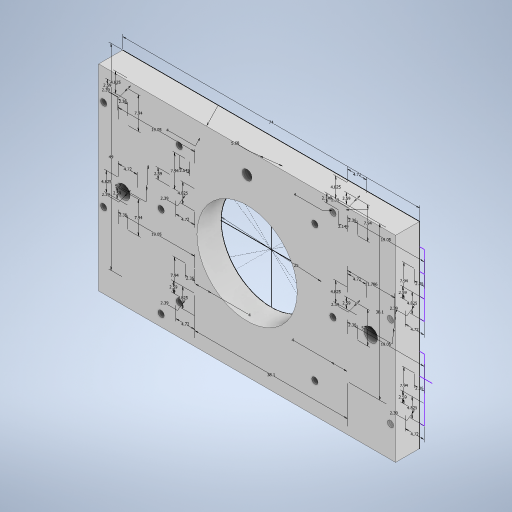
# Autodesk Inventor part: adapter-plate
Saved by Autodesk Inventor 2024 (Build 280153000, 153)
## iProperties
Created: 2023-08-30
Part Number: adapter-plate
Material: Generic
Document SubType Name: Modeling
Designer: raad
Density: 1 g/cm^3
Appearance: Default
Author: raad
Autodesk Inventor part; units mm, degrees
ref_plane "YZ Plane" through (0, 0, 0) normal (1, 0, 0) x (0, 1, 0)
ref_plane "XZ Plane" through (0, 0, 0) normal (0, 1, 0) x (-1, 0, 0)
ref_plane "XY Plane" through (0, 0, 0) normal (0, 0, 1) x (1, 0, 0)
sketch "Sketch1" plane through (0, 0, 0) normal (0, 0, 1) x (1, 0, 0)
  line L0 (37, -24.5) -> (-37, -24.5)
  line L1 (-37, -24.5) -> (-37, 24.5)
  line L2 (-37, 24.5) -> (37, 24.5)
  line L3 (37, 24.5) -> (37, -24.5)
  line L4 (37, -24.5) -> (-37, 24.5) construction
  line L5 (-37, -24.5) -> (37, 24.5) construction
  circle A0 centre (0, 0) radius 12.5
  line L6 (-19.05, 19.05) -> (19.05, 19.05)
  line L7 (19.05, 19.05) -> (19.05, -19.05)
  line L8 (19.05, -19.05) -> (-19.05, -19.05)
  line L9 (-19.05, -19.05) -> (-19.05, 19.05)
  line L10 (-19.05, 19.05) -> (19.05, -19.05) construction
  line L11 (19.05, 19.05) -> (-19.05, -19.05) construction
  line L12 (19.05, 19.05) -> (16.9012, 19.05)
  line L13 (16.9012, 19.05) -> (16.9012, 16.9012)
  line L14 (16.9012, 16.9012) -> (19.05, 16.9012)
  line L15 (19.05, 16.9012) -> (19.05, 19.05)
  line L16 (0, 19.05) -> (0, -19.05)
  line L17 (-19.05, 0) -> (19.05, 0)
  line L18 (-16.9012, 19.05) -> (-16.9012, 16.9012)
  line L19 (-16.9012, 16.9012) -> (-19.05, 16.9012)
  line L20 (19.05, 0) -> (-19.05, 0)
  line L21 (16.9012, -19.05) -> (16.9012, -16.9012)
  line L22 (16.9012, -16.9012) -> (19.05, -16.9012)
  line L23 (-16.9012, -16.9012) -> (-19.05, -16.9012)
  line L24 (-16.9012, -19.05) -> (-16.9012, -16.9012)
  line L25 (19.05, 0) -> (30.8356, 0)
  line L26 (-19.05, 0) -> (-30.8356, 0)
  circle A1 centre (-16.9012, 16.9012) radius 2
  circle A2 centre (16.9012, 16.9012) radius 2
  circle A3 centre (16.9012, -16.9012) radius 2
  circle A4 centre (-16.9012, -16.9012) radius 2
  circle A5 centre (-30.8356, 0) radius 2.85
  circle A6 centre (30.8356, 0) radius 2.85
  line L27 (-30.8356, 14.9012) -> (-30.8356, 2.85)
  line L28 (-38.1003, 8.8756) -> (-19.0503, 8.8756)
  line L29 (-22.8548, 8.8756) -> (-20.3098, 8.8756)
  line L30 (-21.4103, 8.8756) -> (-21.4103, 0.9356)
  line L31 (-38.1719, 10.7443) -> (-35.8119, 10.7443)
  line L32 (-35.7403, 8.8756) -> (-35.7403, 16.8156)
  line L33 (-38.1719, 16.29) -> (-38.1719, 13.7)
  line L34 (-35.7403, 14.2256) -> (-19.0503, 14.2256)
  line L35 (-19.0503, 14.2256) -> (-19.0503, 8.8756)
  line L36 (-25.2148, 0.9356) -> (-25.2148, 3.5256)
  line L37 (-21.4103, 3.5256) -> (-38.1003, 3.5256)
  line L38 (-38.1003, 14.2256) -> (-35.7403, 14.2256)
  line L39 (-21.4103, 3.5256) -> (-19.0503, 3.5256)
  line L40 (-19.0503, 3.5256) -> (-19.0503, 8.8756)
  line L41 (-35.8119, 14.2256) -> (-35.8119, 19.0506)
  line L42 (-38.1003, 19.0506) -> (-33.3803, 19.0506)
  line L43 (-33.3803, 19.0506) -> (-33.3803, 14.2256)
  line L44 (-19.0503, 3.5256) -> (-19.0503, -1.2994)
  line L45 (-19.0503, -1.2994) -> (-23.7703, -1.2994)
  line L46 (-23.7703, -1.2994) -> (-23.7703, 3.5256)
  circle A7 centre (-35.7403, 16.8156) radius 1.195
  circle A8 centre (-21.4103, 0.9356) radius 1.195
  line L47 (30.8356, -2.85) -> (30.8356, -14.9012)
  line L48 (33.9356, -8.8756) -> (40.1, -8.8756)
  line L49 (19.05, -8.8756) -> (38.1, -8.8756)
  line L50 (35.74, -8.8756) -> (35.74, -16.8156)
  line L51 (21.41, -8.8756) -> (21.41, -0.9356)
  line L52 (21.41, -3.5256) -> (38.1, -3.5256)
  line L53 (38.1, -3.5256) -> (38.1, -8.8756)
  line L54 (35.74, -14.2256) -> (19.05, -14.2256)
  line L55 (19.05, -3.5256) -> (21.41, -3.5256)
  line L56 (30.8356, -14.2256) -> (33.1956, -14.2256)
  line L57 (38.1, -14.2256) -> (38.1, -8.8756)
  line L58 (19.05, 1.2994) -> (23.77, 1.2994)
  line L59 (23.77, 1.2994) -> (23.77, -3.5256)
  line L60 (38.1, -14.2256) -> (38.1, -19.0506)
  line L61 (38.1, -19.0506) -> (33.38, -19.0506)
  line L62 (33.38, -19.0506) -> (33.38, -14.2256)
  circle A9 centre (21.41, -0.9356) radius 1.195
  circle A10 centre (35.74, -16.8156) radius 1.195
  line L63 (-38.1, -13.7) -> (-19.05, -13.7)
  line L64 (-21.41, -13.7) -> (-21.41, -21.64)
  line L65 (-35.74, -13.7) -> (-35.74, -5.76)
  line L66 (-35.74, -8.35) -> (-19.05, -8.35)
  line L67 (-19.05, -7.985) -> (-19.05, -13.335)
  line L68 (-21.41, -19.05) -> (-38.1, -19.05)
  line L69 (-38.1, -8.35) -> (-35.74, -8.35)
  line L70 (-21.41, -19.05) -> (-19.05, -19.05)
  line L71 (-19.05, -18.685) -> (-19.05, -13.335)
  line L72 (-38.1, -3.525) -> (-33.38, -3.525)
  line L73 (-33.38, -3.525) -> (-33.38, -8.35)
  line L74 (-19.05, -19.05) -> (-19.05, -23.875)
  line L75 (-19.05, -23.875) -> (-23.77, -23.875)
  line L76 (-23.77, -23.875) -> (-23.77, -19.05)
  circle A11 centre (-35.74, -5.76) radius 1.195
  circle A12 centre (-21.41, -21.64) radius 1.195
  line L77 (19.05, 13.7) -> (38.1, 13.7)
  line L78 (35.74, 13.7) -> (35.74, 5.76)
  line L79 (21.41, 13.7) -> (21.41, 21.64)
  line L80 (21.41, 19.05) -> (38.1, 19.05)
  line L81 (38.1, 19.05) -> (38.1, 13.7)
  line L82 (35.74, 8.35) -> (19.05, 8.35)
  line L83 (19.05, 19.05) -> (21.41, 19.05)
  line L84 (35.74, 8.35) -> (38.1, 8.35)
  line L85 (38.1, 8.35) -> (38.1, 13.7)
  line L86 (19.05, 23.875) -> (23.77, 23.875)
  line L87 (23.77, 23.875) -> (23.77, 19.05)
  line L88 (38.1, 8.35) -> (38.1, 3.525)
  line L89 (38.1, 3.525) -> (33.38, 3.525)
  line L90 (33.38, 3.525) -> (33.38, 8.35)
  circle A13 centre (21.41, 21.64) radius 1.195
  circle A14 centre (35.74, 5.76) radius 1.195
  arc A15 (-37, 21.2315) -> (-36.9905, 20.9193) centre (-31.8628, 21.2315) ccw
  line L91 (-38.1, -3.525) -> (-38.1, -19.05)
  line L92 (19.05, 1.2994) -> (19.05, -14.2256)
  circle A16 centre (0, 19.05) radius 2.84
  dimension "d29" = 5.7
  dimension "d0" = 74
  dimension "d1" = 49
  dimension "d2" = 25
  dimension "d3" = 38.1
  dimension "d4" = 38.1
  dimension "d5" = 2.1488
  dimension "d6" = 2.1488
  dimension "d7" = 11.7856
  dimension "d24" = 4
  dimension "d25" = 4
  dimension "d26" = 4
  dimension "d27" = 4
  dimension "d28" = 5.7
  dimension "d30" = 19.05
  dimension "d31" = 2.545
  dimension "d32" = 7.94
  dimension "d33" = 2.36
  dimension "d34" = 7.94
  dimension "d35" = 2.59
  dimension "d36" = 2.59
  dimension "d37" = 4.825
  dimension "d39" = 4.825
  dimension "d40" = 4.72
  dimension "d41" = 2.39
  dimension "d42" = 2.39
  dimension "d43" = 19.05
  dimension "d44" = 2.36
  dimension "d45" = 7.94
  dimension "d46" = 2.36
  dimension "d47" = 7.94
  dimension "d48" = 2.59
  dimension "d49" = 2.59
  dimension "d50" = 4.825
  dimension "d51" = 4.72
  dimension "d52" = 4.825
  dimension "d53" = 4.72
  dimension "d54" = 2.39
  dimension "d55" = 2.39
  dimension "d56" = 19.05
  dimension "d57" = 2.36
  dimension "d58" = 7.94
  dimension "d59" = 2.36
  dimension "d60" = 7.94
  dimension "d61" = 2.59
  dimension "d62" = 2.59
  dimension "d63" = 4.825
  dimension "d64" = 4.72
  dimension "d65" = 4.825
  dimension "d66" = 4.72
  dimension "d67" = 2.39
  dimension "d68" = 2.39
  dimension "d69" = 19.05
  dimension "d70" = 2.36
  dimension "d71" = 7.94
  dimension "d72" = 2.36
  dimension "d73" = 7.94
  dimension "d74" = 2.59
  dimension "d75" = 2.59
  dimension "d76" = 4.825
  dimension "d77" = 4.72
  dimension "d78" = 4.825
  dimension "d79" = 4.72
  dimension "d80" = 2.39
  dimension "d81" = 2.39
  constraints: 186 end point, 32 point on line, 30 perpendicular, 16 centre point, 16 coincident, 13 symmetric about line, 11 parallel, 8 midpoint, 4 horizontal, 3 vertical, 2 point on circle, 1 tangent, 1 vertical alignment, 2 other
  measures "d0" distance of L1.end L2.end
  measures "d1" distance of L0.end L1.end
  measures "d2" diameter of A0
  measures "d3" distance of L7.end L8.end
  measures "d4" distance of L6.end L7.end
  measures "d5" distance of L14.end L13.end
  measures "d6" distance of L13.end L12.end
  measures "d7" distance of L20.start L25.end
  measures "d24" diameter of A1
  measures "d25" diameter of A2
  measures "d26" diameter of A3
  measures "d27" diameter of A4
  measures "d28" diameter of A5
  measures "d30" distance of L28.start L28.end
  measures "d31" distance of L29.start L29.end
  measures "d32" distance of L30.start L30.end
  measures "d33" distance of L31.start L31.end
  measures "d34" distance of L32.start L32.end
  measures "d35" distance of L33.start L33.end
  measures "d36" distance of L36.start L36.end
  measures "d37" distance of L41.start L41.end
  measures "d39" distance of L39.end L44.end
  measures "d40" distance of L44.end L45.end
  measures "d41" diameter of A7
  measures "d42" diameter of A8
  measures "d43" distance of L49.start L53.end
  measures "d44" distance of L53.end L50.start
  measures "d45" distance of L50.start L50.end
  measures "d46" distance of L49.start L51.start
  measures "d47" distance of L51.start L51.end
  measures "d48" distance of L51.end L52.start
  measures "d49" distance of L50.end L54.start
  measures "d50" distance of L55.start L58.start
  measures "d51" distance of L58.start L58.end
  measures "d52" distance of L57.start L60.end
  measures "d53" distance of L60.end L61.end
  measures "d54" diameter of A9
  measures "d55" diameter of A10
  measures "d56" distance of L63.start L63.end
  measures "d57" distance of L63.end L64.start
  measures "d58" distance of L64.start L64.end
  measures "d59" distance of L63.start L65.start
  measures "d60" distance of L65.start L65.end
  measures "d61" distance of L65.end L66.start
  measures "d62" distance of L64.end L68.start
  measures "d63" distance of L69.start L72.start
  measures "d64" distance of L72.start L72.end
  measures "d65" distance of L74.start L74.end
  measures "d66" distance of L74.end L75.end
  measures "d67" diameter of A11
  measures "d68" diameter of A12
  measures "d69" distance of L77.start L81.end
  measures "d70" distance of L81.end L78.start
  measures "d71" distance of L78.start L78.end
  measures "d72" distance of L77.start L79.start
  measures "d73" distance of L79.start L79.end
  measures "d74" distance of L79.end L80.start
  measures "d75" distance of L78.end L82.start
  measures "d76" distance of L83.start L86.start
  measures "d77" distance of L86.start L86.end
  measures "d78" distance of L85.start L88.end
  measures "d79" distance of L88.end L89.end
  measures "d80" diameter of A13
  measures "d81" diameter of A14
extrude "Extrusion1" add sketch "Sketch1" along normal blind 6 contours L0 L1 L68 L76 L75 L74 L8 L7 L54 L62 L61 L3 | A10 | L61 L62 L54 L50 L48 L3 | L1 L63 L64 L68 | L48 L49 L47 L52 L3 | L1 L69 L65 L63 | A12 | L68 L70 L74 L75 L76 | L52 L47 A6 L25 L59 L58 L7 L82 L90 L89 L3 | L50 L54 L47 L49 L48 | A11 | L1 L72 L73 L66 L69 | L65 L66 L9 L63 | L64 L63 L9 L70 | A14 | L89 L90 L82 L84 L3 | L52 L59 L25 A6 L47 | L47 L49 L51 L52 | L1 L37 L27 A5 L26 L46 L45 L9 L66 L73 L72 | L9 L23 A4 L24 L8 | L84 L78 L77 L3 | A6 | L47 L54 L7 L49 | L52 L51 A9 L25 L59 | L1 L28 L27 L37 | L9 L17 A0 L16 L8 L24 A4 L23 | L77 L79 L80 L3 | L82 L7 L77 L78 | L49 L7 L55 L51 | L55 L7 L25 A9 L51 | L25 A9 L7 L58 L59 | L7 L22 A3 L21 L8 L16 A0 L17 | L1 L38 L32 L28 | L37 L46 L26 A5 L27 | L27 L28 L30 L37 | A4 L23 L24 | L24 L23 A4 | A13 | L80 L83 L6 A16 L9 L34 L43 L42 L1 L2 L3 | L7 L17 A0 L16 A16 L6 L13 A2 L14 | A9 L25 | L25 A9 | L7 L8 L21 A3 L22 | L32 L34 L27 L28 | L27 L34 L9 L28 | A5 | L77 L7 L83 L79 | A3 L21 L22 | L22 L21 A3 | L1 L42 L41 A7 L38 | L38 L41 A7 L32 | L32 A7 L41 L42 L43 L34 | L37 L30 A8 L26 L46 | L45 L46 L26 A8 L9 | L17 L9 L19 A1 L18 L6 A16 L16 A0 | L14 A2 L13 L6 L7 | A7 L41 | L28 L9 L39 L30 | L39 L9 L26 A8 L30 | A2 L13 L14 | L14 L13 A2 | A7 L41 | L9 L6 L18 A1 L19 | A8 L26 | L26 A8 | A16 L6 L16 | L16 L6 A16 | A1 L18 L19 | L19 L18 A1 | L6 A16
hole "Hole1" at (-16.9012, -16.9012, 0) at (16.9012, -16.9012, 0) at (16.9012, 16.9012, 0) at (-16.9012, 16.9012, 0) direction (0, 0, 1) diameter 1.567 end through all thread size "M2x0.4" class "6H" standard "ISO Metric profile"
hole "Hole2" at (-30.8356, 0, 0) at (30.8356, 0, 0) direction (0, 0, 1) diameter 3.4 end through all clearance for "Socket Head Cap Screw" size "M3" standard "Ansi Metric M Profile"
hole "Hole3" at (-35.7403, 16.8156, 0) at (-21.4103, 0.9356, 0) at (-35.74, -5.76, 0) at (-21.41, -21.64, 0) at (35.74, -16.8156, 0) at (21.41, -0.9356, 0) at (35.74, 5.76, 0) at (21.41, 21.64, 0) direction (0, 0, 1) diameter 1.567 end through all thread size "M2x0.4" class "6H" standard "ISO Metric profile"
hole "Hole4" at (0, 19.05, 0) direction (0, 0, 1) diameter 2.459 end through all thread size "M3x0.5" class "6H" standard "ISO Metric profile"
body "Solid1"
